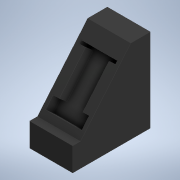
# Autodesk Inventor part: cabinet
Saved by Autodesk Inventor 2020 (Build 240168000, 168)
## iProperties
Created: 2021-03-06
Part Number: cabinet
Material: Generic
Document SubType Name: Modeling
Designer: Harry
Density: 1 g/cm^3
Appearance: Rubber - Black
Author: Harry
Autodesk Inventor part; units mm, degrees
ref_plane "YZ Plane" through (0, 0, 0) normal (1, 0, 0) x (0, 1, 0)
ref_plane "XZ Plane" through (0, 0, 0) normal (0, 1, 0) x (-1, 0, 0)
ref_plane "XY Plane" through (0, 0, 0) normal (0, 0, 1) x (1, 0, 0)
sketch "Sketch1" plane through (0, 0, 0) normal (1, 0, 0) x (0, 1, 0)
  line L0 (0, 0) -> (766.0444, -642.7876)
  line L1 (0, 0) -> (1000, 0) construction
  line L2 (0, 0) -> (0, 100)
  line L3 (0, 100) -> (-300, 100)
  line L4 (-300, 100) -> (-300, -642.7876)
  line L5 (-300, -642.7876) -> (-300, -892.7876)
  line L6 (-300, -892.7876) -> (766.0444, -892.7876)
  line L7 (766.0444, -892.7876) -> (766.0444, -642.7876)
  dimension "d0" = 1000
  dimension "d1" = 40
  dimension "d2" = 100
  dimension "d3" = 300
  dimension "d8" = 250
  constraints: 16 end point, 2 parallel, 1 equal length, 1 horizontal, 1 perpendicular, 1 vertical
  measures "d0" distance of L0.start L0.end
  measures "d1" angle of L0 L1
  measures "d2" distance of L0.start L2.end
  measures "d3" distance of L2.end L3.end
  measures "d8" distance of L4.end L5.end
extrude "Extrusion1" add sketch "Sketch1" against normal blind 550
sketch "Sketch3" plane through (-550, 766.0444, -642.7876) normal (0, 0.6427876, 0.7660444) x (1, 0, 0)
  line L0 (0, -1000) -> (0, 0) projected
  line L1 (550, 0) -> (550, -1000) projected
  line L2 (0, 0) -> (550, -1000) construction
  line L3 (550, -1000) -> (0, -1000) projected
  line L4 (0, -1000) -> (550, 0) construction
  line L5 (125, -760) -> (125, -240)
  line L6 (425, -240) -> (425, -760)
  line L7 (425, -760) -> (125, -240) construction
  line L8 (125, -760) -> (425, -240) construction
  line L9 (425, -240) -> (505, -240) construction
  line L10 (45, -240) -> (45, -200)
  line L11 (45, -200) -> (505, -200)
  line L12 (505, -200) -> (505, -240)
  line L13 (425, -760) -> (505, -760) construction
  line L14 (45, -760) -> (45, -800)
  line L15 (505, -800) -> (505, -760)
  line L16 (505, -760) -> (425, -760)
  line L17 (125, -760) -> (45, -760)
  line L18 (125, -240) -> (132, -240)
  line L19 (418, -240) -> (425, -240)
  line L20 (505, -240) -> (418, -240)
  line L21 (132, -240) -> (45, -240)
  line L22 (505, -800) -> (505, -910)
  line L23 (505, -910) -> (45, -910)
  line L24 (45, -910) -> (45, -800)
  point P0 (275, -500)
  dimension "d9" = 300
  dimension "d10" = 520
  dimension "d11" = 80
  dimension "d12" = 460
  dimension "d13" = 40
  dimension "d14" = 80
  dimension "d15" = 460
  dimension "d16" = 40
  dimension "d21" = 110
  constraints: 44 end point, 6 horizontal, 6 parallel, 4 midpoint, 4 perpendicular, 2 point on line
  measures "d9" distance of L5.end L6.start
  measures "d10" distance of L5.start L5.end
  measures "d11" distance of L6.start L9.end
  measures "d12" distance of L10.end L11.end
  measures "d13" distance of L10.start L10.end
  measures "d14" distance of L6.end L13.end
  measures "d15" distance of L15.start L14.end
  measures "d16" distance of L14.end L14.start
  measures "d21" distance of L22.start L22.end
extrude "Extrusion3" cut sketch "Sketch3" against normal blind 130
body "Solid1"
